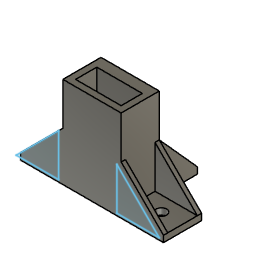
stopka trzymacza v3 (Autodesk Fusion 360 design; units mm, degrees)
Autodesk Fusion 360 part; units mm, degrees
note: some values were not read from the file. Chosen so that the rebuilt part matches the saved one: which bodies a step acts on; which face or edge a step refers to.
sketch "Szkic1" plane through (0, 0, 0) normal (0, 0, 1) x (1, 0, 0)
  line L0 (-20, 15) -> (1.5, 15)
  line L1 (1.5, 15) -> (1.5, 5)
  line L2 (1.5, 5) -> (-20, 5)
  line L3 (-20, 5) -> (-20, 15)
  line L4 (-23, 18) -> (4.5, 18)
  line L5 (4.5, 18) -> (4.5, 2)
  line L6 (4.5, 2) -> (-23, 2)
  line L7 (-23, 2) -> (-23, 18)
  line L8 (-43, 18) -> (24.5, 18)
  line L9 (24.5, 18) -> (24.5, 2)
  line L10 (24.5, 2) -> (-43, 2)
  line L11 (-43, 2) -> (-43, 18)
  line L12 (-23, 18) -> (4, 18)
  line L13 (4, 18) -> (4, 38)
  line L14 (4, 38) -> (-23, 38)
  line L15 (-23, 38) -> (-23, 18)
  dimension "d1" = 21.5
  dimension "d2" = 10
  dimension "d3" = 3
  dimension "d4" = 3
  dimension "d5" = 3
  dimension "d6" = 3
  dimension "d7" = 20
  dimension "d8" = 20
  constraint horizontal L0
  constraint vertical L1
  constraint horizontal L2
  constraint vertical L3
  constraint horizontal L4
  constraint vertical L5
  constraint horizontal L6
  constraint vertical L7
  constraint horizontal L8
  constraint vertical L9
  constraint horizontal L10
  constraint vertical L11
  constraint horizontal L12
  constraint vertical L13
  constraint horizontal L14
  constraint vertical L15
  measures "d1" distance of L0.start L0.end
  measures "d2" distance of L0.start L2.end
  measures "d3" distance of L3 L7
  measures "d4" distance of L1 L5
  measures "d5" distance of L2 L6
  measures "d6" distance of L0 L4
  measures "d7" distance of L7 L11
  measures "d8" distance of L5 L9
extrude "Wyciągnięcie proste4" add sketch "Szkic1" along normal blind 3 contours L4 L8 L12 L13 L14 L15 | L7 L8 L10 L11 | L5 L8 L9 L10 makes body 1 at (-36.3333, 12.6667, 0) makes body 1 at (-14, 31.3333, 0) makes body 2 at (17.8333, 7.3333, 0)
extrude "Wyciągnięcie proste5" add sketch "Szkic1" along normal blind 30 contours L4 L5 L6 L7 L8 L10 L12 bodies 1 2
extrude "Extrude6" add 1 faces at (-12.8333, 3, 30) along direction (0, 0, 1) blind 10 on bodies 1 bodies 1
extrude "Extrude7" add 1 faces at (-12.8333, 3, 40) along direction (0, 0, 1) blind 3 on bodies 1 bodies 1
sketch "Sketch2" plane through (0, 0, 0) normal (0, 1, 0) x (1, 0, 0)
  line L0 (-43, -3) -> (-23, -23)
  line L1 (-23, -23) -> (-23, -3)
  line L2 (-23, -3) -> (-43, -3)
  line L3 (24.5, -3) -> (4.5, -23)
  line L4 (4.5, -23) -> (4.5, -3)
  line L5 (4.5, -3) -> (24.5, -3)
  dimension "d23" = 135
  constraint vertical L1
  constraint perpendicular L1 L2
  constraint parallel L1 L4
  constraint perpendicular L4 L5
  measures "d23" angle of L2 L3
extrude "Extrude8" add sketch "Sketch2" along normal blind 2 from surface at 2 contours L0 L1 L2 bodies 1
extrude "Extrude9" add sketch "Sketch2" along normal blind 2 from surface at 2 contours L3 L4 L5 bodies 1
extrude "Extrude10" add 1 faces at (4, 24.6667, 1) along direction (1, 0, 0) blind 0.5 on bodies 1 bodies 1
extrude "Extrude11" add 1 faces at (11.1667, 18, 1) along direction (0, 1, 0) blind 2 on bodies 1 bodies 1
extrude "Extrude12" add sketch "Sketch2" along normal blind 2 from surface at 18 contours L3 L4 L5 bodies 1
extrude "Extrude13" add sketch "Sketch2" along normal blind 2 from surface at 18 separate body contours L0 L1 L2 makes body 3
extrude "Extrude14" add 1 faces at (-36.3333, 18, 1) along direction (0, 1, 0) blind 2 on bodies 1 bodies 1 3
extrude "Extrude15" add 1 faces at (-13.8333, 18, 16.3333) along direction (0, 1, 0) blind 2 on bodies 1 bodies 1
sketch "Sketch3" plane through (4.5, 0, 0) normal (1, 0, 0) x (0, 1, 0)
  line L0 (20, 3) -> (20, 0)
  line L1 (20, 0) -> (38, 0)
  line L2 (38, 0) -> (38, 3)
  line L3 (38, 3) -> (20, 3)
  line L4 (20, 23) -> (38, 3)
  line L5 (20, 3) -> (20, 23)
  constraint coincident L2.end L3.start
  constraint coincident L0.start L3.end
sketch "Sketch4" plane through (-23, 0, 0) normal (-1, 0, 0) x (0, -1, 0)
  line L0 (-20, 0) -> (-20, 3)
  line L1 (-20, 3) -> (-38, 3)
  line L2 (-38, 3) -> (-38, 0)
  line L3 (-38, 0) -> (-20, 0)
  line L4 (-38, 3) -> (-20, 3)
  line L5 (-20, 23) -> (-38, 3)
  line L6 (-20, 23) -> (-20, 3)
  constraint coincident L1.end L2.start
  constraint coincident L0.end L1.start
  constraint vertical L6
extrude "Extrude16" add sketch "Sketch3" against normal blind 2 contours L3 L4 L5 bodies 1
extrude "Extrude17" add sketch "Sketch4" against normal blind 2 contours L1 L4 L5 L6 bodies 1
sketch "Sketch5" plane through (0, 0, 3) normal (0, 0, 1) x (-1, 0, 0)
  line L0 (-24.5, -18) -> (-4.5, -18)
  line L1 (-4.5, -18) -> (-4.5, -4)
  line L2 (-4.5, -4) -> (-24.5, -4)
  line L3 (-24.5, -4) -> (-24.5, -18)
  circle A0 centre (-14.5, -11) radius 2.5
  circle A1 centre (33, -11) radius 2.5
  line L4 (23, -2) -> (23, -20)
  circle A2 centre (9.25, -29) radius 2.5
  line L5 (21, -38) -> (21, -20)
  line L6 (21, -38) -> (-2.5, -38)
  dimension "d48" = 5
  dimension "d49" = 7
  dimension "d50" = 5
  dimension "d51" = 10
  dimension "d52" = 10
  dimension "d53" = 5
  dimension "d54" = 11.75
  dimension "d55" = 9
  measures "d48" diameter of A0
  measures "d49" distance of L0 A0.centre
  measures "d50" diameter of A1
  measures "d51" distance of A1.centre L4
  measures "d52" distance of L1 A0.centre
  measures "d53" diameter of A2
  measures "d54" distance of A2.centre L5
  measures "d55" distance of A2.centre L6
extrude "Extrude18" cut sketch "Sketch5" against normal blind 8 contours A0 | A1 | A2 bodies 1
equation "d23 = 180 deg - 45 deg"
equation "d34 = 14.00 mm + 4 mm"
equation "d37 = 14.00 mm + 4 mm"
equation "d54 = ( 23.5 / 2 ) * 1 mm"
